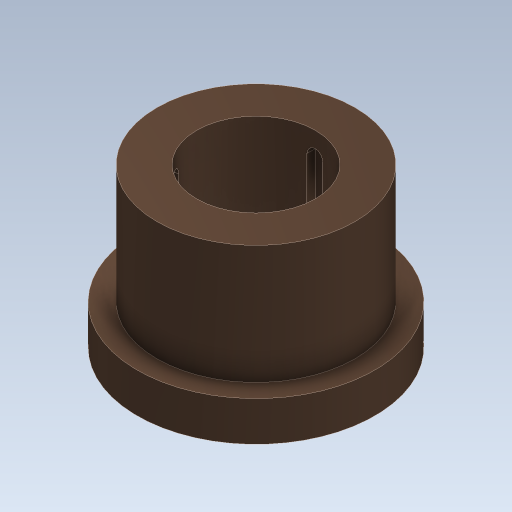
# Autodesk Inventor part: Pump-Motor-CW-Rotation:Bush
Saved by Autodesk Inventor 2024.2 (Build 282272000, 272)
## iProperties
Created: 2025-06-16
Material: Bronze, Soft Tin
Document SubType Name: Modeling
Density: 8.874 g/cm^3
Appearance: Bronze - Satin
Designer: cw
Author: cw
Autodesk Inventor part; units mm, degrees
ref_plane "YZ Plane" through (0, 0, 0) normal (1, 0, 0) x (0, 1, 0)
ref_plane "XY Plane" through (0, 0, 0) normal (0, 0, 1) x (1, 0, 0)
sketch "Sketch1" plane through (0, 0, 0) normal (0, 1, 0) x (-1, 0, 0)
  line L0 (0, 0) -> (15, 0)
  line L1 (15, 0) -> (15, 20)
  line L2 (15, 20) -> (0, 20)
  line L3 (0, 20) -> (0, 0)
  line L4 (12.5, 20) -> (12.5, 5)
  line L5 (12.5, 5) -> (15, 5)
  line L6 (7.5, 20) -> (7.5, 0)
  dimension "d1" = 30
  dimension "d2" = 25
  dimension "d3" = 15
  dimension "d4" = 5
  dimension "d5" = 15
  constraints: 14 end point, 3 perpendicular, 2 midpoint, 2 parallel, 2 point on line, 1 horizontal, 1 vertical
  measures "d1" diameter of L1 L3
  measures "d2" diameter of L4 L3
  measures "d3" distance between parallel lines of L2 L5
  measures "d4" distance between parallel lines of L0 L5
  measures "d5" diameter of L6 L3
revolve "Revolution1" add sketch "Sketch1" angle 360 about axis through (0, 0, 20) along (0, 0, -1) contours L6 L2 L4 L5 L1 L0
ref_plane "Work Plane1" through (0, 8.5, 0) normal (0, 1, 0) x (-1, 0, 0)
sketch "Sketch2" plane through (0, 8.5, 0) normal (0, 1, 0) x (-1, 0, 0)
  line L0 (0, 18) -> (0, 2) construction
  line L1 (1, 17) -> (1, 3)
  line L2 (-1, 3) -> (-1, 17)
  arc A0 (1, 17) -> (-1, 17) centre (0, 17) ccw
  arc A1 (-1, 3) -> (1, 3) centre (0, 3) ccw
  line L3 (-12.5, 20) -> (12.5, 20) construction
  point P0 (0, 0)
  point P1 (0, 10)
  point P2 (0, 18)
  dimension "d8" = 16
  dimension "d9" = 2
  dimension "d10" = 2
  constraints: 8 end point, 7 point on circle, 4 tangent, 2 centre point, 2 point on line, 1 midpoint, 1 parallel, 1 vertical, 1 vertical alignment
  measures "d8" distance of L0.start L0.end
  measures "d9" distance between parallel lines of L2 L1
  measures "d10" distance from line of point (0, 18) L3
extrude "Extrusion1" cut sketch "Sketch2" against normal up to surface
pattern_circular "Circular Pattern1" count 3 over 360 about axis through (0, 0, -10) along (0, 0, 1) of "Extrusion1"
body "Solid1"
